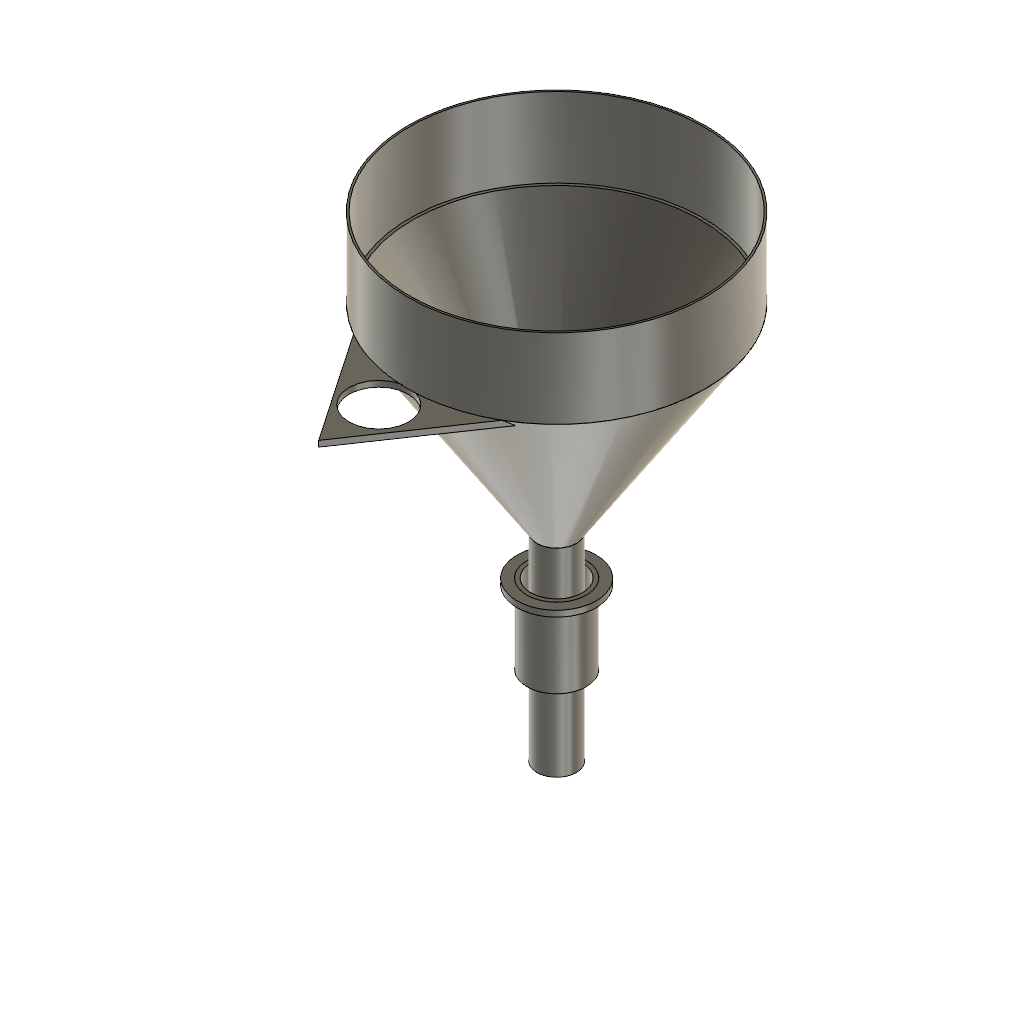
LN2-Funnel (Autodesk Fusion 360 design; units mm, degrees)
part number: 2026-09-08-10-13-18-004
Autodesk Fusion 360 part; units mm, degrees
sketch "Skizze1" plane through (0, 0, 0) normal (0, 0, 1) x (1, 0, 0)
  circle A0 centre (0, 0) radius 15
  dimension "d1" = 30
  constraint coincident A0.centre origin
  measures "d1" diameter of A0
extrude "Extrusion1" add sketch "Skizze1" along normal blind 40 makes body 1
hole "Bohrung1" at (0, 0, 40) direction (0, 0, -1) diameter 26 depth 40 tip angle 180 bodies 1
sketch "Skizze2" plane through (0, 0, 0) normal (0, 0, 1) x (1, 0, 0)
move_face "Fläche verschieben1" to x (1, 0, 0) y (0, 1, 0) z (0, 0, 1) at (0, 0, -40) 1 faces at (14.9814, -0.7477, 26.6667) on bodies 1
sketch "Skizze3" plane through (0, 0, 40) normal (0, 0, 1) x (-1, 0, 0)
  circle A0 centre (0, 0) radius 13
  circle A1 centre (0, 0) radius 15
  circle A2 centre (0, 0) radius 20
  dimension "d8" = 40
  constraint coincident A0.centre A1.centre
  measures "d8" diameter of A2
extrude "Extrusion2" add sketch "Skizze3" along normal blind 3 separate body contours A2 makes body 2
move_body "Verschieben1" bodies 2 to x (1, 0, 0) y (0, 1, 0) z (0, 0, 1) at (0, 0, -3)
move_body "Verschieben2" bodies 1 2 to x (1, 0, 0) y (0, 1, 0) z (0, 0, 1) at (0, 100, 0)
sketch "Skizze4" plane through (0, 0, 0) normal (0, 0, 1) x (1, 0, 0)
  circle A0 centre (0, 0) radius 10
  dimension "d11" = 20
  constraint coincident A0.centre origin
  measures "d11" diameter of A0
extrude "Extrusion3" add sketch "Skizze4" along normal blind 100 separate body makes body 3
hole "Bohrung2" at (0, 0, 100) direction (0, 0, -1) diameter 16 depth 100 tip angle 180 bodies 3
sketch "Skizze5" plane through (0, 0, 0) normal (0, 0, 1) x (1, 0, 0)
  line L0 (0, 0) -> (69.999, 0)
  line L1 (69.999, 0) -> (69.999, -20)
  line L2 (69.999, -20) -> (0, -20)
  line L3 (0, -20) -> (0, 0)
  dimension "d23" = 20
  constraint horizontal L0
  constraint vertical L1
  constraint horizontal L2
  constraint vertical L3
  constraint coincident L0.start L3.end
  measures "d23" distance of L0.start L2.end
move_body "Verschieben4" bodies 1 2 to x (1, 0, 0) y (0, 1, 0) z (0, 0, 1) at (0, -100, 40)
sketch "Skizze6" plane through (0, 0, 0) normal (1, 0, 0) x (0, 1, 0)
sketch "Skizze9" plane through (0, 0, 0) normal (0, 1, 0) x (1, 0, 0)
  circle A0 centre (0, -30) radius 1.5
  dimension "d37" = 3
  measures "d37" diameter of A0
extrude "Extrusion6" add sketch "Skizze9" along normal blind 3.5 separate body makes body 4
move_body "Verschieben9" bodies 4 to x (1, 0, 0) y (0, 1, 0) z (0, 0, 1) at (0, 9.7, 30)
copy_body "Körper kopieren/einfügen1" bodies 4 makes body 5
move_body "Verschieben10" bodies 5 to x (0.719677, 0.691766, -0.059362) y (-0.691766, 0.707107, -0.146491) z (-0.059362, 0.146491, 0.987429) at (17.5813, -20.8555, 3.7231)
copy_body "Körper kopieren/einfügen2" bodies 5 makes body 6
move_body "Verschieben11" bodies 6 to x (0.932191, 0.234969, -0.275335) y (-0.25539, 0.965998, -0.04029) z (0.256506, 0.107876, 0.960504) at (-31.5838, 2.4301, 2.6956)
move_body "Verschieben12" bodies 5 to x (0.967275, 0.061841, -0.246077) y (-0.09035, 0.990221, -0.106297) z (0.237097, 0.125051, 0.963404) at (-11.6093, -10.8101, 2.7885)
copy_body "Körper kopieren/einfügen3" bodies 4 makes body 7
move_body "Verschieben13" bodies 7 to x (1, 0, 0) y (0, 1, 0) z (0, 0, 1) at (0, -22.9, 0)
move_body "Verschieben14" bodies 7 to x (0.547058, -0.826381, -0.1335) y (0.834484, 0.550958, 0.009061) z (0.066065, -0.116361, 0.991007) at (-3.8594, 6.7024, 0.7599)
copy_body "Körper kopieren/einfügen4" bodies 7 makes body 8
move_body "Verschieben15" bodies 8 to x (1, 0, 0) y (0, 1, 0) z (0, 0, 1) at (19.7277, 11.7192, 0.4711)
copy_body "Körper kopieren/einfügen5" bodies 4 makes body 9
move_body "Verschieben16" bodies 9 to x (1, 0, 0) y (0, 1, 0) z (0, 0, 1) at (0, -23, 0)
extrude "Extrusion7" add 1 faces at (9.2886, -0.6961, 100) along direction (0, 0, 1) blind 100 draft 33 separate body on bodies 3 makes body 10
ref_plane "Arbeitsebene2" through (0, 0, 197) normal (0, 0, 1) x (1, 0, 0)
sketch "Skizze11" plane through (0, 0, 197) normal (0, 0, 1) x (1, 0, 0)
  circle A0 centre (0, 0) radius 72.9925
  line L0 (40.1544, -60.9552) -> (0, -120)
  line L1 (0, -120) -> (-40.2621, -60.8841)
  constraint coincident A0 L0.start
  constraint coincident A0 L1.end
shell "Schale1" thickness 2 removed faces 1 at (-6.6684, -16.9909, 200) on bodies 10
extrude "Extrusion8" add sketch "Skizze11" along normal blind 3 contours A0 L0 L1 bodies 10
hole "Bohrung7" at (-0.4068, -89.2145, 200) direction (0, 0, -1) diameter 30 depth 3 tip angle 180 bodies 10
hole "Bohrung6" at (0, 0, 0) direction (0, 0, 1) diameter 16 end through all bodies 10
ref_plane "Arbeitsebene3" through (-0.0254, -22.5094, 200) normal (0, 0, 1) x (1, 0, 0)
sketch "Skizze12" plane through (0, 0, 200) normal (0, 0, 1) x (1, 0, 0)
  circle A0 centre (0, 0) radius 75
  dimension "d55" = 150
  constraint coincident A0.centre origin
  measures "d55" diameter of A0
extrude "Extrusion9" add sketch "Skizze12" along normal blind 40 separate body makes body 11
hole "Bohrung8" at (0, 0, 240) direction (0, 0, -1) diameter 148 depth 40 tip angle 180 bodies 11
named bodies: "Kragen", "Kragenkranz", "Tunnel", "Verbindungsstück 3", "Verbindungsstück 1", "Verbindungsstück 4", "Verbindungsstück 5", "Verbindungsstück 2", "Verbindungsstück 6", "Trichter", "Kranz"
